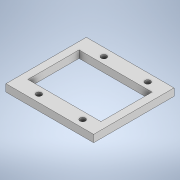
# Autodesk Inventor part: Eyepiece Mount
Saved by Autodesk Inventor 2022 (Build 260153000, 153)
## iProperties
Created: 2023-09-18
Part Number: Eyepiece Mount
Material: Generic
Document SubType Name: Modeling
Designer: fouad
Density: 1 g/cm^3
Appearance: Default
Author: fouad
Autodesk Inventor part; units mm, degrees
ref_plane "YZ Plane" through (0, 0, 0) normal (1, 0, 0) x (0, 1, 0)
ref_plane "XZ Plane" through (0, 0, 0) normal (0, 1, 0) x (-1, 0, 0)
ref_plane "XY Plane" through (0, 0, 0) normal (0, 0, 1) x (1, 0, 0)
sketch "Sketch1" plane through (0, 0, 0) normal (0, 1, 0) x (-1, 0, 0)
  line L0 (4.5, 5.5) -> (-7.5, 5.5)
  line L1 (-7.5, 5.5) -> (-7.5, -5.5)
  line L2 (-7.5, -5.5) -> (4.5, -5.5)
  line L3 (4.5, -5.5) -> (4.5, 5.5)
  line L4 (3.5, 3.5) -> (-6.5, 3.5)
  line L5 (-6.5, 3.5) -> (-6.5, -3.5)
  line L6 (-6.5, -3.5) -> (3.5, -3.5)
  line L7 (3.5, -3.5) -> (3.5, 3.5)
  circle A0 centre (1, 4.5) radius 0.375
  circle A1 centre (1, -4.4) radius 0.375
  circle A2 centre (-5, 4.5) radius 0.375
  circle A3 centre (-5, -4.4) radius 0.375
  point P0 (0, 0)
  dimension "d0" = 12
  dimension "d1" = 11
  dimension "d2" = 5.5
  dimension "d3" = 7.5
  dimension "d4" = 10
  dimension "d5" = 7
  dimension "d6" = 2
  dimension "d7" = 1
  dimension "d8" = 0.75
  dimension "d9" = 3.5
  dimension "d10" = 1
  dimension "d13" = 8.9
  dimension "d16" = 6
  constraints: 16 end point, 4 centre point, 4 parallel, 3 horizontal, 2 perpendicular, 1 vertical, 6 other
  measures "d0" distance of L2.end L1.end
  measures "d1" distance of L1.end L0.end
  measures "d2" distance from line of point (0, 0) L0
  measures "d3" distance from line of point (0, 0) L1
  measures "d4" distance of L6.end L5.end
  measures "d5" distance of L5.end L4.end
  measures "d6" distance between parallel lines of L0 L4
  measures "d7" distance between parallel lines of L3 L7
  measures "d8" diameter of A0
  measures "d9" distance from line of L3 A0.centre
  measures "d10" distance from line of L0 A0.centre
  measures "d13" distance of A0.centre A1.centre
  measures "d16" distance of A0.centre A2.centre
extrude "Extrusion1" add sketch "Sketch1" along normal blind 1
body "Solid1"
